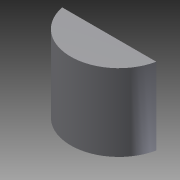
# Autodesk Inventor part: X_Belt_Shoe
Saved by Autodesk Inventor 2012 (Build 160160000, 160)
## iProperties
Created: 2012-07-05
Part Number: X_Belt_Shoe
Material: Default
Document SubType Name: Modeling
Designer: Administrator
Density: 1 g/cm^3
Author: Administrator
Autodesk Inventor part; units mm, degrees
ref_plane "YZ Plane" through (0, 0, 0) normal (1, 0, 0) x (0, 1, 0)
ref_plane "XZ Plane" through (0, 0, 0) normal (0, 1, 0) x (-1, 0, 0)
ref_plane "XY Plane" through (0, 0, 0) normal (0, 0, 1) x (1, 0, 0)
sketch "Sketch1" plane through (0, 0, 0) normal (0, 0, 1) x (1, 0, 0)
  circle A0 centre (0, 0) radius 5
  line L0 (-4.899, -1) -> (4.899, -1)
  dimension "d0" = 10
  dimension "d3" = 4
  constraints: 2 end point, 2 point on circle, 1 centre point, 1 coincident, 1 horizontal
  measures "d0" diameter of A0
  measures "d3" distance edge to line of A0 L0
extrude "Extrusion2" add sketch "Sketch1" along normal blind 8 contours L0 A0 picked at (0.432, -3.4521)
sketch "Sketch3" plane through (-4.899, -1, 0) normal (0, 1, 0) x (1, 0, 0)
  line L0 (9.798, 0) -> (9.798, -8) projected
  line L1 (9.798, 0) -> (0, 0) projected
  circle A0 centre (4.899, -4) radius 2
  point P0 (4.899, 0)
  point P1 (4.899, 0)
  point P2 (9.798, -4)
  dimension "d6" = 4
  constraints: 2 midpoint, 1 centre point, 1 horizontal alignment, 1 vertical alignment
  measures "d6" diameter of A0
extrude "Extrusion3" cut sketch "Sketch3" against normal blind 2
body "Solid2"
